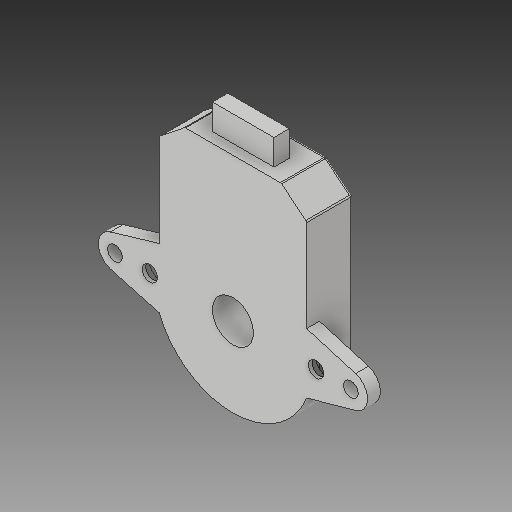
# Autodesk Inventor part: AMT102-V
Saved by Autodesk Inventor 2019 (Build 230136000, 136)
## iProperties
Created: 2018-09-21
Part Number: AMT102-V
Material: 一般
Document SubType Name: Modeling
Designer: Kyohei
Density: 1 g/cm^3
Appearance: 既定
Mass: 10.4709 g
Surface Area: 42.5793 cm^2
Volume: 10.4709 cm^3
Author: Kyohei
Autodesk Inventor part; units mm, degrees
ref_plane "YZ Plane" through (0, 0, 0) normal (1, 0, 0) x (0, 1, 0)
ref_plane "XZ Plane" through (0, 0, 0) normal (0, 1, 0) x (-1, 0, 0)
ref_plane "XY Plane" through (0, 0, 0) normal (0, 0, 1) x (1, 0, 0)
sketch "スケッチ1" plane through (0, 0, 0) normal (0, 0, 1) x (1, 0, 0)
  line L0 (0, 0) -> (-28.77, 0)
  line L1 (-28.77, 0) -> (-28.77, -33.8125)
  line L2 (-28.77, -33.8125) -> (0, -33.8125)
  line L3 (0, -33.8125) -> (0, 0)
  circle A0 centre (-14.385, -28.04) radius 15.5
  line L4 (0, -4) -> (-5, 0)
  line L5 (-23.77, 0) -> (-28.77, -4)
  dimension "d0" = 28.77
  dimension "d2" = 31
  dimension "d4" = 4
  dimension "d5" = 4
  dimension "d6" = 5
  dimension "d7" = 5
  dimension "d66" = 28.04
  constraints: 12 end point, 4 point on line, 2 parallel, 2 point on circle, 1 centre point, 1 horizontal, 1 perpendicular
  measures "d0" distance of L2.end L1.end
  measures "d2" diameter of A0
  measures "d4" distance from line of L4.start L0
  measures "d5" distance from line of L5.end L0
  measures "d6" distance from line of L4.end L3
  measures "d7" distance from line of L1 L5.start
  measures "d66" distance from line of A0.centre L0
extrude "押し出し1" add sketch "スケッチ1" along normal blind 9 contours L4 L3 A0 L1 L5 L0 | L3 L2 L1 A0 | A0 L2
sketch "スケッチ2" plane through (0, 0, 9) normal (0, 0, 1) x (1, 0, 0)
  line L0 (-5, 0) -> (-23.77, 0) projected
  arc A0 (-28.77, -33.8125) -> (0, -33.8125) centre (-14.385, -28.04) ccw projected
  point P0 (0, 0)
  constraints: 1 coincident
hole "穴1" at (-14.385, -28.04, 9) direction (0, 0, -1) diameter 8 end through all
sketch "スケッチ3" plane through (0, 0, 9) normal (0, 0, 1) x (1, 0, 0)
  line L0 (-28.77, -33.8125) -> (-38.2682, -31.1712)
  line L1 (-28.77, -22.086) -> (-38.3232, -24.9246)
  circle A0 centre (-37.3975, -28.04) radius 3.25
  circle A1 centre (-14.385, -28.04) radius 4 projected
  line L2 (0, -33.8125) -> (9.4982, -31.1712)
  line L3 (0, -22.086) -> (9.5532, -24.9246)
  circle A2 centre (8.6275, -28.04) radius 3.25
  line L4 (-28.77, -4) -> (-28.77, -33.8125) projected
  line L5 (0, -33.8125) -> (0, -4) projected
  point P0 (0, 0)
  dimension "d19" = 5.954
  dimension "d20" = 6.5
  dimension "d53" = 46.025
  dimension "d54" = 23.0125
  dimension "d55" = 6.5
  constraints: 8 end point, 4 point on circle, 4 tangent, 3 horizontal alignment, 2 centre point, 2 point on line, 1 coincident
  measures "d19" vertical distance of L1.start point (-14.385, -28.04)
  measures "d20" diameter of A0
  measures "d53" distance of A2.centre A0.centre
  measures "d54" distance of A2.centre A1.centre
  measures "d55" diameter of A2
extrude "押し出し2" add sketch "スケッチ3" against normal blind 2.5 contours L0 A0 L1 L4 | A0 | L5 L3 A2 L2 | A2
sketch "スケッチ4" plane through (0, 0, 6.5) normal (0, 0, -1) x (-1, 0, 0)
  arc A0 (0, -33.8125) -> (28.77, -33.8125) centre (14.385, -28.04) ccw projected
  point P0 (0, 0)
  point P1 (30.6, -28.04)
  point P2 (-1.83, -28.04)
  dimension "d26" = 16.215
  dimension "d27" = 16.215
  constraints: 2 horizontal alignment
  measures "d26" distance of point (30.6, -28.04) A0.centre
  measures "d27" distance of point (-1.83, -28.04) A0.centre
hole "穴2" at (-30.6, -28.04, 6.5) at (1.83, -28.04, 6.5) direction (0, 0, 1) diameter 3 end through all
sketch "スケッチ5" plane through (0, 0, 6.5) normal (0, 0, -1) x (-1, 0, 0)
  circle A0 centre (30.6, -28.04) radius 1.5 projected
  circle A1 centre (-1.83, -28.04) radius 1.5 projected
  point P0 (0, 0)
  constraints: 2 coincident
hole "穴3" at (-30.6, -28.04, 6.5) at (1.83, -28.04, 6.5) direction (0, 0, 1) diameter 5.6 depth 1.8
sketch "スケッチ6" plane through (0, 0, 6.5) normal (0, 0, -1) x (-1, 0, 0)
  circle A0 centre (14.385, -28.04) radius 4 projected
  point P0 (0, 0)
  point P1 (37.3975, -28.04)
  point P2 (-8.6275, -28.04)
  dimension "d43" = 23.0125
  dimension "d45" = 23.0125
  constraints: 4 horizontal alignment, 1 coincident
  measures "d43" distance of point (37.398, -28.04) A0.centre
  measures "d45" distance of point (-8.627, -28.04) point (14.385, -28.04)
hole "穴4" at (-37.3975, -28.04, 6.5) at (8.6275, -28.04, 6.5) at (-14.385, -28.04, 6.5) direction (0, 0, 1) diameter 2.87 end through all
fillet "フィレット1" radius 0.4 4 edges at (-28.77, -4, 4.5) (-23.77, 0, 4.5) (-5, 0, 4.5) (0, -4, 4.5)
fillet "フィレット2" radius 0.5 10 edges at (-28.7305, -4.019, 0) (-26.2497, -1.9838, 0) (-23.7621, -0.0225, 0) (-14.385, 0, 0) (-5.0079, -0.0225, 0) (-2.5203, -1.9838, 0) (-0.0395, -4.019, 0) (0, -19.0024, 0) (-28.77, -19.0024, 0) (-14.385, -43.54, 0)
sketch "スケッチ7" plane through (-23.6297, 0, 9) normal (0, 1, 0) x (1, 0, 0)
  line L0 (3.2447, 5) -> (15.2447, 5)
  line L1 (15.2447, 5) -> (15.2447, 2)
  line L2 (15.2447, 2) -> (3.2447, 2)
  line L3 (3.2447, 2) -> (3.2447, 5)
  line L4 (18.4894, 0) -> (0, 0) projected
  point P0 (23.6297, 9)
  dimension "d60" = 3
  dimension "d61" = 12
  dimension "d62" = 8.385
  dimension "d63" = 2
  constraints: 8 end point, 2 parallel, 1 horizontal, 1 perpendicular
  measures "d60" distance of L2.end L0.start
  measures "d61" distance of L0.start L0.end
  measures "d62" distance from line of L1 point (23.63, 9)
  measures "d63" distance between parallel lines of L4 L2
extrude "押し出し3" add sketch "スケッチ7" along normal blind 5
equation "\"d4\" = d5"
equation "\"d6\" = d7"
equation "\"d54\" = 0.5 * d53"
equation "\"d55\" = d20"
equation "\"d27\" = d26"
equation "\"d45\" = d43"
equation "\"d62\" = -0.5 * d61 + 0.5 * d0"
